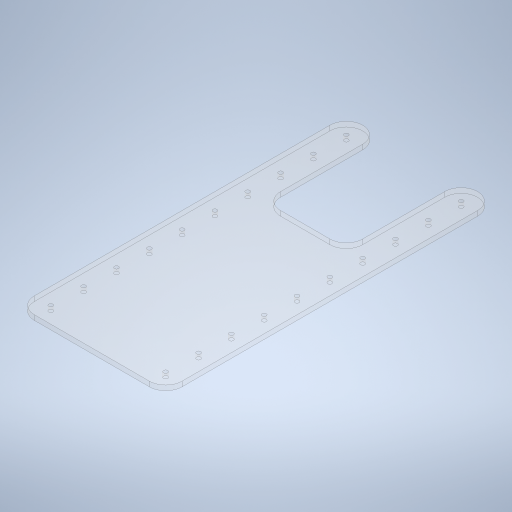
# Autodesk Inventor part: ElectronicsBaseplateV01
Saved by Autodesk Inventor 2023 (Build 270158000, 158)
## iProperties
Created: 2022-11-08
Part Number: ElectronicsBaseplateV01
Material: Polycarbonate, Clear
Document SubType Name: Modeling
Designer: Administrator
Density: 1.2 g/cm^3
Appearance: Polycarbonate - Clear
Author: Administrator
Autodesk Inventor part; units mm, degrees
ref_plane "YZ Plane" through (0, 0, 0) normal (1, 0, 0) x (0, 1, 0)
ref_plane "XZ Plane" through (0, 0, 0) normal (0, 1, 0) x (-1, 0, 0)
ref_plane "XY Plane" through (0, 0, 0) normal (0, 0, 1) x (1, 0, 0)
sketch "Sketch1" plane through (0, 0, 0) normal (0, 1, 0) x (-1, 0, 0)
  line L0 (10, 0) -> (80, 0)
  line L1 (90, -10) -> (90, -190)
  line L2 (80, -200) -> (80, -200)
  line L3 (0, -190) -> (0, -10)
  arc A0 (90, -10) -> (80, 0) centre (80, -10) ccw
  arc A1 (0, -190) -> (10, -200) centre (10, -190) ccw
  arc A2 (80, -200) -> (90, -190) centre (80, -190) ccw
  arc A3 (10, 0) -> (0, -10) centre (10, -10) ccw
  circle A4 centre (80, -10) radius 1.25
  circle A5 centre (80, -30) radius 1.25
  circle A6 centre (80, -50) radius 1.25
  circle A7 centre (80, -70) radius 1.25
  circle A8 centre (80, -90) radius 1.25
  circle A9 centre (80, -110) radius 1.25
  circle A10 centre (80, -130) radius 1.25
  circle A11 centre (80, -150) radius 1.25
  circle A12 centre (80, -170) radius 1.25
  circle A13 centre (80, -190) radius 1.25
  circle A14 centre (10, -10) radius 1.25
  circle A15 centre (10, -30) radius 1.25
  circle A16 centre (10, -50) radius 1.25
  circle A17 centre (10, -70) radius 1.25
  circle A18 centre (10, -90) radius 1.25
  circle A19 centre (10, -110) radius 1.25
  circle A20 centre (10, -130) radius 1.25
  circle A21 centre (10, -150) radius 1.25
  circle A22 centre (10, -170) radius 1.25
  circle A23 centre (10, -190) radius 1.25
  line L4 (20, -190) -> (20, -140)
  line L5 (30, -130) -> (60, -130)
  line L6 (70, -140) -> (70, -190)
  arc A24 (70, -190) -> (80, -200) centre (80, -190) ccw
  line L7 (10, -200) -> (10, -200)
  arc A25 (70, -140) -> (60, -130) centre (60, -140) ccw
  arc A26 (30, -130) -> (20, -140) centre (30, -140) ccw
  arc A27 (10, -200) -> (20, -190) centre (10, -190) ccw
  point P0 (0, 0)
  point P1 (90, -200)
  point P2 (90, 0)
  point P3 (0, -200)
  point P4 (20, -200)
  point P5 (10, -200)
  dimension "d0" = 90
  dimension "d1" = 200
  dimension "d15" = 10
  dimension "d16" = 2.5
  dimension "d19" = 20
  dimension "d24" = 2.5
  dimension "d27" = 20
  dimension "d35" = 10
  dimension "d36" = 10
  constraints: 28 centre point, 16 end point, 16 point on circle, 16 tangent, 12 point on line, 5 equal radius, 3 perpendicular, 3 vertical, 2 coincident, 2 horizontal, 2 parallel, 36 other
  measures "d0" distance of point (90, -200) point (0, -200)
  measures "d1" distance of point (90, 0) point (90, -200)
  measures "d15" radius of A0
  measures "d16" diameter of A4
  measures "d19" distance of A4.centre A5.centre
  measures "d24" diameter of A14
  measures "d27" distance of A14.centre A15.centre
  measures "d35" radius of A24
  measures "d36" radius of A25
extrude "Extrusion2" add sketch "Sketch1" along normal blind 3
body "Solid2"
